Autodesk Inventor part; units mm, degrees
(part 2 of 2)
sketch "Sketch18" plane through (0, 0, -0.2) normal (0, 0, -1) x (-1, 0, 0)
  line L0 (-13.9597, 17.5749) -> (-9.7521, 15.1456) projected
  line L1 (-9.7521, 15.1456) -> (-5.5444, 17.5749) projected
  line L2 (-5.5444, 17.5749) -> (-5.5444, 22.4335) projected
  line L3 (-5.5444, 22.4335) -> (-9.7521, 24.8628) projected
  line L4 (-9.7521, 24.8628) -> (-13.9597, 22.4335) projected
  line L5 (-13.9597, 22.4335) -> (-13.9597, 17.5749) projected
  line L6 (-34.8886, 65.4022) -> (-34.8886, 72.3894) projected
  line L7 (-34.8886, 72.3894) -> (-40.9397, 75.883) projected
  line L8 (-40.9397, 75.883) -> (-46.9908, 72.3894) projected
  line L9 (-46.9908, 72.3894) -> (-46.9908, 65.4022) projected
  line L10 (-46.9908, 65.4022) -> (-40.9397, 61.9086) projected
  line L11 (-40.9397, 61.9086) -> (-34.8886, 65.4022) projected
  line L12 (-49.5403, 66.4665) -> (-49.5403, 71.3251) projected
  line L13 (-49.5403, 71.3251) -> (-53.7479, 73.7544) projected
  line L14 (-53.7479, 73.7544) -> (-57.9556, 71.3251) projected
  line L15 (-57.9556, 71.3251) -> (-57.9556, 66.4665) projected
  line L16 (-57.9556, 66.4665) -> (-53.7479, 64.0372) projected
  line L17 (-53.7479, 64.0372) -> (-49.5403, 66.4665) projected
  line L18 (0, 0) -> (-63.5, 0)
  line L19 (-63.5, 0) -> (-63.5, 88.9)
  line L20 (-63.5, 88.9) -> (0, 88.9)
  line L21 (0, 88.9) -> (0, 0)
  line L22 (-40.9397, 26.9914) -> (-46.9908, 23.4978) projected
  line L23 (-46.9908, 23.4978) -> (-46.9908, 16.5106) projected
  line L24 (-46.9908, 16.5106) -> (-40.9397, 13.017) projected
  line L25 (-40.9397, 13.017) -> (-34.8886, 16.5106) projected
  line L26 (-34.8886, 16.5106) -> (-34.8886, 23.4978) projected
  line L27 (-34.8886, 23.4978) -> (-40.9397, 26.9914) projected
  line L28 (-22.5603, 13.017) -> (-16.5092, 16.5106) projected
  line L29 (-16.5092, 16.5106) -> (-16.5092, 23.4978) projected
  line L30 (-16.5092, 23.4978) -> (-22.5603, 26.9914) projected
  line L31 (-22.5603, 26.9914) -> (-28.6114, 23.4978) projected
  line L32 (-28.6114, 23.4978) -> (-28.6114, 16.5106) projected
  line L33 (-28.6114, 16.5106) -> (-22.5603, 13.017) projected
  line L34 (-24.4329, 66.1976) -> (-24.4329, 72.4542) projected
  line L35 (-22.5603, 61.9086) -> (-16.5092, 65.4022) projected
  line L36 (-16.5092, 65.4022) -> (-16.5092, 72.3894) projected
  line L37 (-16.5092, 72.3894) -> (-22.5603, 75.883) projected
  line L38 (-22.5603, 75.883) -> (-28.6114, 72.3894) projected
  line L39 (-28.6114, 72.3894) -> (-28.6114, 65.4022) projected
  line L40 (-28.6114, 65.4022) -> (-22.5603, 61.9086) projected
  line L41 (-41.2436, 50.1475) -> (-41.2436, 57.1347) projected
  line L42 (-41.2436, 57.1347) -> (-47.2947, 60.6283) projected
  line L43 (-47.2947, 60.6283) -> (-53.3458, 57.1347) projected
  line L44 (-53.3458, 57.1347) -> (-53.3458, 50.1475) projected
  line L45 (-53.3458, 50.1475) -> (-47.2947, 46.6539) projected
  line L46 (-47.2947, 46.6539) -> (-41.2436, 50.1475) projected
  line L47 (-31.4992, 48.8078) -> (-25.4481, 52.3014) projected
  line L48 (-25.4481, 52.3014) -> (-25.4481, 59.2887) projected
  line L49 (-25.4481, 59.2887) -> (-31.4992, 62.7823) projected
  line L50 (-31.4992, 62.7823) -> (-37.5503, 59.2887) projected
  line L51 (-37.5503, 59.2887) -> (-37.5503, 52.3014) projected
  line L52 (-37.5503, 52.3014) -> (-31.4992, 48.8078) projected
  line L53 (-31.4992, 26.1177) -> (-25.4481, 29.6113) projected
  line L54 (-25.4481, 29.6113) -> (-25.4481, 36.5986) projected
  line L55 (-25.4481, 36.5986) -> (-31.4992, 40.0922) projected
  line L56 (-31.4992, 40.0922) -> (-37.5503, 36.5986) projected
  line L57 (-37.5503, 36.5986) -> (-37.5503, 29.6113) projected
  line L58 (-37.5503, 29.6113) -> (-31.4992, 26.1177) projected
  line L59 (-47.2947, 28.2717) -> (-41.2436, 31.7653) projected
  line L60 (-41.2436, 31.7653) -> (-41.2436, 38.7525) projected
  line L61 (-41.2436, 38.7525) -> (-47.2947, 42.2461) projected
  line L62 (-47.2947, 42.2461) -> (-53.3458, 38.7525) projected
  line L63 (-53.3458, 38.7525) -> (-53.3458, 31.7653) projected
  line L64 (-53.3458, 31.7653) -> (-47.2947, 28.2717) projected
  line L65 (-22.2564, 31.7653) -> (-16.2053, 28.2717) projected
  line L66 (-16.2053, 28.2717) -> (-10.1542, 31.7653) projected
  line L67 (-10.1542, 31.7653) -> (-10.1542, 38.7525) projected
  line L68 (-10.1542, 38.7525) -> (-16.2053, 42.2461) projected
  line L69 (-16.2053, 42.2461) -> (-22.2564, 38.7525) projected
  line L70 (-22.2564, 38.7525) -> (-22.2564, 31.7653) projected
  line L71 (-22.2564, 50.1475) -> (-16.2053, 46.6539) projected
  line L72 (-16.2053, 46.6539) -> (-10.1542, 50.1475) projected
  line L73 (-10.1542, 50.1475) -> (-10.1542, 57.1347) projected
  line L74 (-10.1542, 57.1347) -> (-16.2053, 60.6283) projected
  line L75 (-16.2053, 60.6283) -> (-22.2564, 57.1347) projected
  line L76 (-22.2564, 57.1347) -> (-22.2564, 50.1475) projected
  spline S0 degree 2 poles (-15.0708, 11.7851) (-14.865, 12.3203) (-14.1322, 12.8554) (-13.5724, 12.8554) knots 0 0 0 0.5 1 1 1 projected
  spline S1 degree 2 poles (-13.5724, 12.8554) (-12.9795, 12.8554) (-12.2468, 12.2873) (-12.0492, 11.7604) knots 0 0 0 0.5 1 1 1 projected
  spline S2 degree 2 poles (-12.0492, 11.7604) (-11.8351, 11.2005) (-11.7034, 9.7679) (-11.7034, 8.6976) knots 0 0 0 0.5 1 1 1 projected
  spline S3 degree 2 poles (-11.7034, 8.6976) (-11.7034, 7.7013) (-11.8516, 6.1205) (-12.0574, 5.6018) knots 0 0 0 0.5 1 1 1 projected
  spline S4 degree 2 poles (-12.0574, 5.6018) (-12.2715, 5.0667) (-13.0042, 4.5315) (-13.5724, 4.5315) knots 0 0 0 0.5 1 1 1 projected
  spline S5 degree 2 poles (-13.5724, 4.5315) (-14.1405, 4.5315) (-14.8568, 5.0667) (-15.0626, 5.5854) knots 0 0 0 0.5 1 1 1 projected
  spline S6 degree 2 poles (-15.0626, 5.5854) (-15.2684, 6.1041) (-15.4331, 7.6437) (-15.4331, 8.6893) knots 0 0 0 0.5 1 1 1 projected
  spline S7 degree 2 poles (-15.4331, 8.6893) (-15.4331, 9.735) (-15.2684, 11.2829) (-15.0708, 11.7851) knots 0 0 0 0.5 1 1 1 projected
  spline S8 degree 2 poles (-13.5724, 13.9834) (-15.2273, 13.9834) (-16.8163, 11.4228) (-16.8163, 8.6893) knots 0 0 0 0.5 1 1 1 projected
  spline S9 degree 2 poles (-16.8163, 8.6893) (-16.8163, 6.0382) (-15.2437, 3.4035) (-13.5724, 3.4035) knots 0 0 0 0.5 1 1 1 projected
  spline S10 degree 2 poles (-13.5724, 3.4035) (-11.9092, 3.4035) (-10.3202, 5.9476) (-10.3202, 8.6976) knots 0 0 0 0.5 1 1 1 projected
  spline S11 degree 2 poles (-10.3202, 8.6976) (-10.3202, 11.3734) (-11.8927, 13.9834) (-13.5724, 13.9834) knots 0 0 0 0.5 1 1 1 projected
  line L77 (-3.6676, 13.7693) -> (-8.6241, 13.7693) projected
  line L78 (-8.6241, 13.7693) -> (-8.6241, 12.7319) projected
  line L79 (-8.6241, 12.7319) -> (-6.821, 12.7319) projected
  line L80 (-6.821, 12.7319) -> (-6.821, 3.5764) projected
  line L81 (-6.821, 3.5764) -> (-5.7671, 3.5764) projected
  spline S12 degree 2 poles (-5.7671, 3.5764) (-5.7012, 4.3998) (-4.7132, 4.9926) (-3.6676, 4.9926) knots 0 0 0 0.5 1 1 1 projected
  line L82 (-3.6676, 4.9926) -> (-3.6676, 5.9229) projected
  line L83 (-3.6676, 5.9229) -> (-5.5119, 5.9229) projected
  line L84 (-5.5119, 5.9229) -> (-5.5119, 12.7319) projected
  line L85 (-5.5119, 12.7319) -> (-3.6676, 12.7319) projected
  line L86 (-3.6676, 12.7319) -> (-3.6676, 13.7693) projected
  line L87 (-59.8324, 75.4752) -> (-54.8759, 75.4752) projected
  line L88 (-54.8759, 75.4752) -> (-54.8759, 76.5126) projected
  line L89 (-54.8759, 76.5126) -> (-56.679, 76.5126) projected
  line L90 (-56.679, 76.5126) -> (-56.679, 85.6682) projected
  line L91 (-56.679, 85.6682) -> (-57.7329, 85.6682) projected
  spline S13 degree 2 poles (-57.7329, 85.6682) (-57.7988, 84.8448) (-58.7868, 84.252) (-59.8324, 84.252) knots 0 0 0 0.5 1 1 1 projected
  line L92 (-59.8324, 84.252) -> (-59.8324, 83.3216) projected
  line L93 (-59.8324, 83.3216) -> (-57.9881, 83.3216) projected
  line L94 (-57.9881, 83.3216) -> (-57.9881, 76.5126) projected
  line L95 (-57.9881, 76.5126) -> (-59.8324, 76.5126) projected
  line L96 (-59.8324, 76.5126) -> (-59.8324, 75.4752) projected
  spline S14 degree 2 poles (-48.4292, 77.4595) (-48.635, 76.9243) (-49.3678, 76.3891) (-49.9276, 76.3891) knots 0 0 0 0.5 1 1 1 projected
  spline S15 degree 2 poles (-49.9276, 76.3891) (-50.5205, 76.3891) (-51.2532, 76.9572) (-51.4508, 77.4842) knots 0 0 0 0.5 1 1 1 projected
  spline S16 degree 2 poles (-51.4508, 77.4842) (-51.6649, 78.044) (-51.7966, 79.4767) (-51.7966, 80.547) knots 0 0 0 0.5 1 1 1 projected
  spline S17 degree 2 poles (-51.7966, 80.547) (-51.7966, 81.5432) (-51.6484, 83.124) (-51.4426, 83.6427) knots 0 0 0 0.5 1 1 1 projected
  spline S18 degree 2 poles (-51.4426, 83.6427) (-51.2285, 84.1779) (-50.4958, 84.7131) (-49.9276, 84.7131) knots 0 0 0 0.5 1 1 1 projected
  spline S19 degree 2 poles (-49.9276, 84.7131) (-49.3595, 84.7131) (-48.6432, 84.1779) (-48.4374, 83.6592) knots 0 0 0 0.5 1 1 1 projected
  spline S20 degree 2 poles (-48.4374, 83.6592) (-48.2316, 83.1405) (-48.0669, 81.6009) (-48.0669, 80.5552) knots 0 0 0 0.5 1 1 1 projected
  spline S21 degree 2 poles (-48.0669, 80.5552) (-48.0669, 79.5096) (-48.2316, 77.9617) (-48.4292, 77.4595) knots 0 0 0 0.5 1 1 1 projected
  spline S22 degree 2 poles (-49.9276, 75.2612) (-48.2727, 75.2612) (-46.6837, 77.8217) (-46.6837, 80.5552) knots 0 0 0 0.5 1 1 1 projected
  spline S23 degree 2 poles (-46.6837, 80.5552) (-46.6837, 83.2064) (-48.2563, 85.8411) (-49.9276, 85.8411) knots 0 0 0 0.5 1 1 1 projected
  spline S24 degree 2 poles (-49.9276, 85.8411) (-51.5908, 85.8411) (-53.1798, 83.2969) (-53.1798, 80.547) knots 0 0 0 0.5 1 1 1 projected
  spline S25 degree 2 poles (-53.1798, 80.547) (-53.1798, 77.8711) (-51.6073, 75.2612) (-49.9276, 75.2612) knots 0 0 0 0.5 1 1 1 projected
  constraints: 8 end point, 2 parallel, 1 horizontal, 1 perpendicular, 26 other
extrude "Extrusion21" add sketch "Sketch18" along normal blind 0.4 bodies 3
fillet "Fillet2" radius 3.175 8 edges at (63.5, 0, 0.2) (63.5, 88.9, 0.2) (0, 0, 0.2) (0, 88.9, 0.2) (63.5, 0, -0.3) (63.5, 88.9, -0.3) (0, 0, -0.3) (0, 88.9, -0.3)
